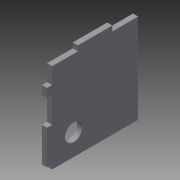
# Autodesk Inventor part: Motor support
Saved by Autodesk Inventor 2015 (Build 190159000, 159)
## iProperties
Created: 2014-08-15
Part Number: Motor support
Material: Generic
Document SubType Name: Modeling
Designer: karl
Density: 1 g/cm^3
Appearance: Default
Author: karl
Autodesk Inventor part; units mm, degrees
ref_plane "YZ Plane" through (0, 0, 0) normal (1, 0, 0) x (0, 1, 0)
ref_plane "XZ Plane" through (0, 0, 0) normal (0, 1, 0) x (-1, 0, 0)
ref_plane "XY Plane" through (0, 0, 0) normal (0, 0, 1) x (1, 0, 0)
sketch "Sketch1" plane through (0, 0, 0) normal (1, 0, 0) x (0, 1, 0)
  line L0 (25, -12.5) -> (-25, -12.5)
  line L1 (-25, -12.5) -> (-25, 50)
  line L2 (-25, 50) -> (25, 50)
  line L3 (25, 50) -> (25, -12.5)
  circle A0 centre (-12.5, 0) radius 12.5 construction
  circle A1 centre (-12.5, 0) radius 5
  point P0 (0, 0)
  point P1 (0, -12.5)
  dimension "d0" = 50
  dimension "d1" = 50
  dimension "d2" = 25
  dimension "d3" = 12.5
  dimension "d4" = 10
  constraints: 8 end point, 2 centre point, 2 parallel, 1 coincident, 1 horizontal, 1 horizontal alignment, 1 midpoint, 1 perpendicular, 1 tangent, 1 vertical alignment
  measures "d0" distance of L0.start L0.end
  measures "d1" distance from line of L2 point (0, 0)
  measures "d2" diameter of A0
  measures "d3" distance from line of L0 point (0, 0)
  measures "d4" diameter of A1
extrude "Extrusion1" add sketch "Sketch1" along normal blind 3
sketch "Sketch2" plane through (0, 0, 0) normal (-1, 0, 0) x (0, 0, 1)
  line L0 (-10, -25) -> (10, -25)
  line L1 (10, -25) -> (10, -28)
  line L2 (10, -28) -> (-10, -28)
  line L3 (-10, -28) -> (-10, -25)
  line L4 (50, -25) -> (-12.5, -25) projected
  line L5 (25, -25) -> (30, -25)
  line L6 (30, -25) -> (30, -28)
  line L7 (30, -28) -> (25, -28)
  line L8 (25, -28) -> (25, -25)
  point P0 (0, 0)
  point P1 (0, -28)
  dimension "d7" = 20
  dimension "d8" = 3
  dimension "d9" = 5
  dimension "d10" = 3
  dimension "d11" = 15
  constraints: 16 end point, 4 parallel, 2 horizontal, 2 perpendicular, 1 collinear, 1 midpoint, 1 point on line, 1 vertical alignment
  measures "d7" distance of L1.end L2.end
  measures "d8" distance of L0.end L1.end
  measures "d9" distance of L6.end L7.end
  measures "d10" distance of L5.end L6.end
  measures "d11" distance between parallel lines of L8 L1
extrude "Extrusion2" add sketch "Sketch2" against normal blind 3
sketch "Sketch3" plane through (0, 0, 0) normal (-1, 0, 0) x (0, 0, 1)
  line L0 (50, -25) -> (47, -25)
  line L1 (47, -25) -> (47, -10)
  line L2 (47, -10) -> (50, -10)
  line L3 (50, -10) -> (50, -25)
  line L4 (50, 25) -> (47, 25)
  line L5 (47, 25) -> (47, 10)
  line L6 (47, 10) -> (50, 10)
  line L7 (50, 10) -> (50, 25)
  point P0 (0, 0)
  dimension "d14" = 20
  dimension "d15" = 10
  dimension "d16" = 3
  constraints: 16 end point, 4 parallel, 2 horizontal, 2 perpendicular, 1 collinear
  measures "d14" distance between parallel lines of L2 L6
  measures "d15" distance from line of point (0, 0) L6
  measures "d16" distance between parallel lines of L7 L5
extrude "Extrusion3" cut sketch "Sketch3" against normal blind 3
sketch "Sketch4" plane through (0, 0, 0) normal (-1, 0, 0) x (0, 0, 1)
  circle A0 centre (0, -12.5) radius 5 projected
  circle A1 centre (0, -4) radius 1.5
  point P0 (0, 0)
  dimension "d19" = 3
  dimension "d20" = 8.5
  constraints: 1 centre point, 1 vertical alignment
  measures "d19" diameter of A1
  measures "d20" distance of A1.centre A0.centre
extrude "Extrusion4" cut sketch "Sketch4" against normal blind 3 contours A1
pattern_circular "Circular Pattern1" count 6 over 360 about axis through (0, -12.5, 0) along (1, 0, 0) of "Extrusion4"
sketch "Sketch5" plane through (0, 0, 0) normal (-1, 0, 0) x (0, 0, 1)
  circle A0 centre (0, -12.5) radius 5 projected
  circle A1 centre (0, -12.5) radius 12.5 construction
  line L0 (12.5, -7.5) -> (15.5, -7.5)
  line L1 (15.5, -7.5) -> (15.5, -17.5)
  line L2 (15.5, -17.5) -> (12.5, -17.5)
  line L3 (12.5, -17.5) -> (12.5, -7.5)
  point P0 (0, 0)
  point P1 (12.5, -12.5)
  dimension "d26" = 25
  dimension "d27" = 3
  dimension "d28" = 10
  constraints: 8 end point, 2 parallel, 1 centre point, 1 coincident, 1 horizontal, 1 horizontal alignment, 1 midpoint, 1 perpendicular, 1 tangent
  measures "d26" diameter of A1
  measures "d27" distance of L1.end L2.end
  measures "d28" distance of L0.end L1.end
extrude "Extrusion5" cut sketch "Sketch5" against normal blind 3 contours L0 L1 L2 L3
equation "\"d15\" = 0.5 * d14"
body "Solid1"
